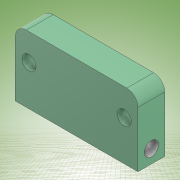
# Autodesk Inventor part: SoporteDerecha
Saved by Autodesk Inventor 2022 (Build 260153000, 153)
## iProperties
Created: 2022-01-31
Part Number: SoporteDerecha
Material: Genérico
Document SubType Name: Modeling
Designer: Marco
Density: 1 g/cm^3
Appearance: Valor por defecto
Author: Marco
Autodesk Inventor part; units mm, degrees
ref_plane "YZ Plane" through (0, 0, 0) normal (1, 0, 0) x (0, 1, 0)
ref_plane "XZ Plane" through (0, 0, 0) normal (0, 1, 0) x (-1, 0, 0)
ref_plane "XY Plane" through (0, 0, 0) normal (0, 0, 1) x (1, 0, 0)
sketch "Boceto1" plane through (0, 0, 0) normal (0, 0, 1) x (1, 0, 0)
  line L0 (0, 0) -> (55, 0)
  line L1 (55, 0) -> (55, 20)
  line L2 (55, 20) -> (0, 20)
  line L3 (0, 20) -> (0, 0)
  circle A0 centre (6.165, 8) radius 3.175
  line L4 (27.5, 20) -> (27.5, 0)
  circle A1 centre (48.835, 8) radius 3.175
  dimension "d0" = 6.35
  dimension "d1" = 55
  dimension "d3" = 20
  dimension "d23" = 42.67
  dimension "d31" = 8
  constraints: 10 end point, 2 centre point, 2 midpoint, 2 parallel, 1 horizontal, 1 perpendicular, 1 symmetric about line, 1 other
  measures "d0" diameter of A0
  measures "d1" distance of L0.end L0.start
  measures "d3" distance of L0.start L2.end
  measures "d23" distance of A1.centre A0.centre
  measures "d31" vertical distance of L0.start A0.centre
extrude "Extrusión1" add sketch "Boceto1" along normal blind 12
fillet "Empalme1" radius 5 2 edges at (55, 20, 6) (0, 20, 6)
sketch "Boceto7" plane through (0, 0, 0) normal (0, -1, 0) x (1, 0, 0)
  line L0 (0, 0) -> (0, 12) projected
  line L1 (0, 12) -> (55, 12) projected
  line L2 (0, 0) -> (55, 0)
  line L3 (55, 0) -> (55, 12)
  line L4 (55, 12) -> (0, 12)
  line L5 (0, 12) -> (0, 0)
  constraints: 8 end point, 2 parallel, 1 horizontal, 1 perpendicular
extrude "Extrusión5" add sketch "Boceto7" along normal blind 10
sketch "Boceto8" plane through (55, 15, 12) normal (1, 0, 0) x (0, 0, -1)
  circle A0 centre (6, -19) radius 3.175
  line L0 (12, -25) -> (0, -25) projected
  line L1 (12, 0) -> (12, -25) projected
  point P0 (12, -15)
  point P1 (6, -25)
  dimension "d26" = 6.35
  dimension "d27" = 6
  constraints: 1 centre point, 1 midpoint, 1 vertical alignment
  measures "d26" diameter of A0
  measures "d27" distance from line of L0 A0.centre
extrude "Extrusión6" cut sketch "Boceto8" against normal blind 55
